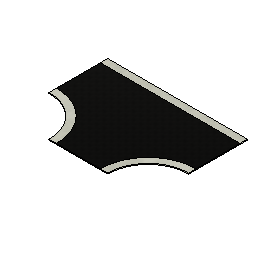
_End Turns - Ruby.568decec-24fa-4051-ab86-487004634091 (Autodesk Fusion 360 design; units mm, degrees)
Autodesk Fusion 360 part; units mm, degrees
sketch "Sketch1" plane through (0, 0, 0) normal (1, 0, 0) x (0, 1, 0)
sketch "Sketch2" plane through (0, 0, 0) normal (0, 0, 1) x (1, 0, 0)
  circle A0 centre (0, 0) radius 660.4
  circle A1 centre (0, 0) radius 1270
  circle A2 centre (-1930.4, 0) radius 660.4
  circle A3 centre (-1930.4, 0) radius 1270
  line L0 (0, 0) -> (0, 1270)
  line L1 (-1930.4, 0) -> (-1930.4, 1270)
  line L2 (0, 1270) -> (-1930.4, 1270)
  line L3 (-1930.4, 1270) -> (-1930.4, 0)
  line L4 (-1930.4, 0) -> (0, 0)
  line L5 (0, 0) -> (0, 1270)
  dimension "d1" = 1320.8
  dimension "d2" = 609.6
  dimension "d3" = 1320.8
  dimension "d4" = 609.6
  constraint coincident A0.centre A1.centre
  constraint tangent A0 A3
  constraint coincident A1 L0.end
  constraint vertical L0
  constraint coincident A2.centre A3.centre
  constraint coincident A3 L1.end
  constraint vertical L1
  constraint horizontal L2
  constraint vertical L3
  constraint horizontal L4
  constraint vertical L5
  measures "d1" diameter of A0
  measures "d3" diameter of A2
extrude "Extrude1" add sketch "Sketch2" against normal blind 12.7 contours A0 A1 A3 L0 L5 | A1 A3 L4 | A1 A3 L2 | A1 A2 A3 L1 L3 picked at (-635.577, 767.3332) picked at (-1062.5692, 59.7006) picked at (-1294.823, 767.3332) makes body 1
sketch "Sketch3" plane through (0, 0, -12.7) normal (0, 0, -1) x (1, 0, 0)
  line L0 (-1930.4, -1270) -> (0, -1270)
  line L1 (0, -1270) -> (0, -660.4)
  arc A0 (-660.4, 0) -> (0, -660.4) centre (0, 0) ccw
  line L2 (-660.4, 0) -> (-1270, 0)
  arc A1 (-1930.4, -660.4) -> (-1270, 0) centre (-1930.4, 0) ccw
  line L3 (-1930.4, -660.4) -> (-1930.4, -1270)
  arc A2 (-549.486, 101.6) -> (101.6, -549.486) centre (0, 0) ccw
  line L4 (101.6, -1371.6) -> (101.6, -549.486)
  line L5 (-2032, -1371.6) -> (101.6, -1371.6)
  line L6 (-2032, -549.486) -> (-2032, -1371.6)
  arc A3 (-2032, -549.486) -> (-1380.914, 101.6) centre (-1930.4, 0) ccw
  line L7 (-549.486, 101.6) -> (-1380.914, 101.6)
  line L8 (-2032, -1371.6) -> (-1930.4, -1371.6)
  line L9 (-1930.4, -1371.6) -> (-1930.4, -470.7354)
  line L10 (-1930.4, -470.7354) -> (-2032, -470.7354)
  line L11 (-2032, -470.7354) -> (-2032, -1371.6)
  line L12 (101.6, -1371.6) -> (0, -1371.6)
  line L13 (0, -1371.6) -> (0, -254)
  line L14 (0, -254) -> (101.6, -254)
  line L15 (101.6, -254) -> (101.6, -1371.6)
  line L16 (-549.486, 101.6) -> (-1862.8596, 101.6)
  line L17 (-1862.8596, 101.6) -> (-1862.8596, 0)
  line L18 (-1862.8596, 0) -> (-549.486, 0)
  line L19 (-549.486, 0) -> (-549.486, 101.6)
  dimension "d7" = 101.6
  constraint horizontal L8
  constraint vertical L9
  constraint horizontal L10
  constraint vertical L11
  constraint horizontal L12
  constraint vertical L13
  constraint horizontal L14
  constraint vertical L15
  constraint horizontal L16
  constraint vertical L17
  constraint horizontal L18
  constraint vertical L19
extrude "Extrude1'" add sketch "Sketch3" against normal blind 12.7 separate body contours L0 L5 L9 L13 | A1 A3 L9 L18 | A0 A2 L13 L18 makes body 2 at (-624.2927, 31.3282, -12.7) makes body 3 at (-1872.5632, 622.3968, -12.7) makes body 4 at (-1286.9333, 1303.8667, -12.7) in component "T"
copy_body "CutPasteBodies1" bodies 1 removing the originals makes body 5 in component "T"
component "T" placed x (1, 0, 0) y (0, 1, 0) z (0, 0, 1) at (0, 0, 0)
